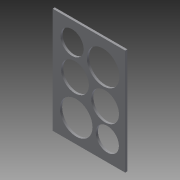
# Autodesk Inventor part: Center
Saved by Autodesk Inventor 2015 (Build 190159000, 159)
## iProperties
Created: 2014-09-15
Part Number: Center
Material: Generic
Document SubType Name: Modeling
Designer: ehagerup
Density: 1 g/cm^3
Appearance: Default
Author: ehagerup
Autodesk Inventor part; units mm, degrees
ref_plane "YZ Plane" through (0, 0, 0) normal (1, 0, 0) x (0, 1, 0)
ref_plane "XZ Plane" through (0, 0, 0) normal (0, 1, 0) x (-1, 0, 0)
ref_plane "XY Plane" through (0, 0, 0) normal (0, 0, 1) x (1, 0, 0)
sketch "Sketch1" plane through (0, 0, 0) normal (0, 1, 0) x (-1, 0, 0)
  circle A0 centre (59.9806, -102.3601) radius 22.5
  circle A1 centre (61.712, -54.745) radius 19.25
  circle A2 centre (65.7506, -15.2725) radius 16
  circle A3 centre (22.7676, -23.4976) radius 22.5
  circle A4 centre (20.1892, -68.6854) radius 19.25
  circle A5 centre (17.0449, -106.5008) radius 16
  line L0 (-7.557, 11.8403) -> (92.5214, 11.8403)
  line L1 (92.5214, 11.8403) -> (92.5214, -134.0855)
  line L2 (92.5214, -134.0855) -> (-7.557, -134.0855)
  line L3 (-7.557, -134.0855) -> (-7.557, 11.8403)
  point P0 (0, 0)
  constraints: 8 end point, 6 centre point, 2 parallel, 1 horizontal, 1 perpendicular
extrude "Extrusion1" add sketch "Sketch1" along normal blind 3
body "Solid1"
